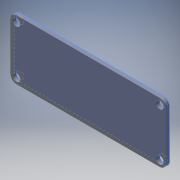
# Autodesk Inventor part: I6ABreakout
Saved by Autodesk Inventor 2018 (Build 220112000, 112)
## iProperties
Created: 2017-11-10
Part Number: I6ABreakout
Material: Generic
Document SubType Name: Modeling
Designer: lsullivan
Density: 1 g/cm^3
Appearance: Default
Author: lsullivan
Autodesk Inventor part; units mm, degrees
ref_plane "YZ Plane" through (0, 0, 0) normal (1, 0, 0) x (0, 1, 0)
ref_plane "XZ Plane" through (0, 0, 0) normal (0, 1, 0) x (-1, 0, 0)
ref_plane "XY Plane" through (0, 0, 0) normal (0, 0, 1) x (1, 0, 0)
sketch "Sketch1" plane through (0, 0, 0) normal (0, 0, 1) x (1, 0, 0)
  line L0 (0, 0) -> (82.55, 0)
  line L1 (82.55, 0) -> (82.55, 31.75)
  line L2 (82.55, 31.75) -> (0, 31.75)
  line L3 (0, 31.75) -> (0, 0)
  dimension "d0" = 82.55
  dimension "d1" = 31.75
  constraints: 8 end point, 2 parallel, 1 horizontal, 1 perpendicular
  measures "d0" distance of L2.end L1.end
  measures "d1" distance of L1.end L0.end
extrude "Extrusion1" add sketch "Sketch1" along normal blind 2
fillet "Fillet1" radius 3.175 1 edges at (0, 31.75, 1)
fillet "Fillet2" radius 3.175 1 edges at (82.55, 31.75, 1)
fillet "Fillet3" radius 3.175 1 edges at (82.55, 0, 1)
fillet "Fillet4" radius 3.175 1 edges at (0, 0, 1)
sketch "Sketch2" plane through (0, 0, 2) normal (0, 0, 1) x (1, 0, 0)
  circle A0 centre (3.175, 3.175) radius 2.032
  arc A1 (0, 3.175) -> (3.175, 0) centre (3.175, 3.175) ccw projected
  line L0 (3.175, 0) -> (79.375, 0) projected
  arc A2 (79.375, 0) -> (82.55, 3.175) centre (79.375, 3.175) ccw projected
  line L1 (82.55, 3.175) -> (82.55, 28.575) projected
  arc A3 (82.55, 28.575) -> (79.375, 31.75) centre (79.375, 28.575) ccw projected
  line L2 (79.375, 31.75) -> (3.175, 31.75) projected
  arc A4 (3.175, 31.75) -> (0, 28.575) centre (3.175, 28.575) ccw projected
  line L3 (0, 28.575) -> (0, 3.175) projected
  point P0 (0, 0)
  dimension "d8" = 4.064
  dimension "d23" = 25.4
  dimension "d25" = 76.2
  constraints: 1 centre point
  measures "d8" diameter of A0
  measures "d23" distance of A4.centre A0.centre
  measures "d25" distance of A2.centre A0.centre
hole "Hole1" at (3.175, 3.175, 2) direction (0, 0, -1) diameter 4.064 end through all
sketch "Sketch7" plane through (0, 0, 2) normal (0, 0, 1) x (1, 0, 0)
  circle A0 centre (3.175, 3.175) radius 2.032 projected
  circle A1 centre (3.175, 3.175) radius 2.032 projected
  arc A2 (0, 3.175) -> (3.175, 0) centre (3.175, 3.175) ccw projected
  line L0 (3.175, 0) -> (79.375, 0) projected
  arc A3 (79.375, 0) -> (82.55, 3.175) centre (79.375, 3.175) ccw projected
  line L1 (82.55, 3.175) -> (82.55, 28.575) projected
  arc A4 (82.55, 28.575) -> (79.375, 31.75) centre (79.375, 28.575) ccw projected
  line L2 (79.375, 31.75) -> (3.175, 31.75) projected
  arc A5 (3.175, 31.75) -> (0, 28.575) centre (3.175, 28.575) ccw projected
  line L3 (0, 28.575) -> (0, 3.175) projected
  circle A6 centre (3.175, 28.575) radius 2.032
  point P0 (0, 0)
  dimension "d28" = 4.064
  constraints: 1 centre point, 1 coincident
  measures "d28" diameter of A6
hole "Hole2" at (3.175, 28.575, 2) direction (0, 0, -1) diameter 4.064 end through all
sketch "Sketch8" plane through (0, 0, 2) normal (0, 0, 1) x (1, 0, 0)
  circle A0 centre (3.175, 3.175) radius 2.032 projected
  circle A1 centre (3.175, 28.575) radius 2.032 projected
  circle A2 centre (3.175, 3.175) radius 2.032 projected
  arc A3 (0, 3.175) -> (3.175, 0) centre (3.175, 3.175) ccw projected
  line L0 (3.175, 0) -> (79.375, 0) projected
  arc A4 (79.375, 0) -> (82.55, 3.175) centre (79.375, 3.175) ccw projected
  line L1 (82.55, 3.175) -> (82.55, 28.575) projected
  arc A5 (82.55, 28.575) -> (79.375, 31.75) centre (79.375, 28.575) ccw projected
  line L2 (79.375, 31.75) -> (3.175, 31.75) projected
  arc A6 (3.175, 31.75) -> (0, 28.575) centre (3.175, 28.575) ccw projected
  line L3 (0, 28.575) -> (0, 3.175) projected
  circle A7 centre (79.375, 28.575) radius 2.032
  point P0 (0, 0)
  dimension "d36" = 4.064
  constraints: 1 centre point, 1 coincident
  measures "d36" diameter of A7
hole "Hole3" at (79.375, 28.575, 2) direction (0, 0, -1) diameter 4.064 end through all
sketch "Sketch9" plane through (0, 0, 2) normal (0, 0, 1) x (1, 0, 0)
  circle A0 centre (3.175, 3.175) radius 2.032 projected
  circle A1 centre (79.375, 28.575) radius 2.032 projected
  circle A2 centre (3.175, 28.575) radius 2.032 projected
  circle A3 centre (3.175, 3.175) radius 2.032 projected
  arc A4 (0, 3.175) -> (3.175, 0) centre (3.175, 3.175) ccw projected
  line L0 (3.175, 0) -> (79.375, 0) projected
  arc A5 (79.375, 0) -> (82.55, 3.175) centre (79.375, 3.175) ccw projected
  line L1 (82.55, 3.175) -> (82.55, 28.575) projected
  arc A6 (82.55, 28.575) -> (79.375, 31.75) centre (79.375, 28.575) ccw projected
  line L2 (79.375, 31.75) -> (3.175, 31.75) projected
  arc A7 (3.175, 31.75) -> (0, 28.575) centre (3.175, 28.575) ccw projected
  line L3 (0, 28.575) -> (0, 3.175) projected
  circle A8 centre (79.375, 3.175) radius 2.032
  point P0 (0, 0)
  dimension "d44" = 4.064
  constraints: 1 centre point, 1 coincident
  measures "d44" diameter of A8
hole "Hole4" at (79.375, 3.175, 2) direction (0, 0, -1) diameter 4.064 end through all
body "Solid1"
